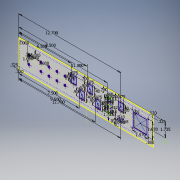
# Autodesk Inventor part: nmt_frontpanel
Saved by Autodesk Inventor 2017 (Build 210142000, 142)
## iProperties
Created: 2017-02-06
Part Number: nmt_frontpanel
Material: Generic
Document SubType Name: Modeling
Designer: Zara
Density: 1 g/cm^3
Appearance: Default
Author: Zara
Autodesk Inventor part; units mm, degrees
ref_plane "YZ Plane" through (0, 0, 0) normal (1, 0, 0) x (0, 1, 0)
ref_plane "XZ Plane" through (0, 0, 0) normal (0, 1, 0) x (-1, 0, 0)
ref_plane "XY Plane" through (0, 0, 0) normal (0, 0, 1) x (1, 0, 0)
sketch "Sketch1" plane through (0, 0, 0) normal (0, 0, 1) x (1, 0, 0)
  line L0 (-212.471, -44.069) -> (212.471, -44.069)
  line L1 (212.471, -44.069) -> (212.471, 44.069)
  line L2 (212.471, 44.069) -> (-212.471, 44.069)
  line L3 (-212.471, 44.069) -> (-212.471, -44.069)
  line L4 (-212.471, -44.069) -> (212.471, 44.069) construction
  line L5 (212.471, -44.069) -> (-212.471, 44.069) construction
  point P0 (0, 0)
  dimension "d0" = 424.942
  dimension "d1" = 88.138
  constraints: 12 end point, 2 midpoint, 2 parallel, 1 horizontal, 1 perpendicular
  measures "d0" distance of L1.end L2.end
  measures "d1" distance of L0.end L1.end
extrude "Extrusion1" add sketch "Sketch1" along normal blind 1.651
sketch "SMA" plane through (0, 0, 1.651) normal (0, 0, 1) x (1, 0, 0)
  line L0 (-209.423, -35.814) -> (209.423, -35.814) construction
  line L1 (209.423, -35.814) -> (209.423, 35.814) construction
  line L2 (209.423, 35.814) -> (-209.423, 35.814) construction
  line L3 (-209.423, 35.814) -> (-209.423, -35.814) construction
  line L4 (212.471, 44.069) -> (-212.471, 44.069) construction
  line L5 (212.471, -44.069) -> (212.471, 44.069) construction
  line L6 (-212.471, 44.069) -> (-212.471, -44.069) projected
  line L7 (-212.471, -44.069) -> (212.471, -44.069) projected
  line L8 (-222.5982, 0) -> (228.0899, 0) construction
  line L9 (0, 79.8165) -> (0, -88.5526) construction
  line L10 (-181.2798, 19.5533) -> (-181.2798, 0.2592) construction
  line L11 (-189.2532, 10.414) -> (-170.7489, 10.414) construction
  arc A0 (-184.023, 8.669) -> (-184.023, 12.159) centre (-181.2798, 10.414) ccw
  line L12 (-184.023, 12.159) -> (-184.023, 8.669)
  line L13 (-145.923, 12.159) -> (-145.923, 8.669)
  arc A1 (-145.923, 8.669) -> (-145.923, 12.159) centre (-143.1798, 10.414) ccw
  line L14 (-184.023, -13.241) -> (-184.023, -16.731)
  arc A2 (-184.023, -16.731) -> (-184.023, -13.241) centre (-181.2798, -14.986) ccw
  line L15 (-145.923, -13.241) -> (-145.923, -16.731)
  arc A3 (-145.923, -16.731) -> (-145.923, -13.241) centre (-143.1798, -14.986) ccw
  line L16 (-120.523, 12.159) -> (-120.523, 8.669)
  arc A4 (-120.523, 8.669) -> (-120.523, 12.159) centre (-117.7798, 10.414) ccw
  arc A5 (-120.523, -16.731) -> (-120.523, -13.241) centre (-117.7798, -14.986) ccw
  line L17 (-120.523, -13.241) -> (-120.523, -16.731)
  line L18 (-95.123, 12.159) -> (-95.123, 8.669)
  arc A6 (-95.123, 8.669) -> (-95.123, 12.159) centre (-92.3798, 10.414) ccw
  arc A7 (-95.123, -16.731) -> (-95.123, -13.241) centre (-92.3798, -14.986) ccw
  line L19 (-95.123, -13.241) -> (-95.123, -16.731)
  line L20 (-69.723, 12.159) -> (-69.723, 8.669)
  arc A8 (-69.723, 8.669) -> (-69.723, 12.159) centre (-66.9798, 10.414) ccw
  arc A9 (-69.723, -16.731) -> (-69.723, -13.241) centre (-66.9798, -14.986) ccw
  line L21 (-69.723, -13.241) -> (-69.723, -16.731)
  point P0 (0, 0)
  point P1 (-178.0286, 10.414)
  point P2 (-139.9286, 10.414)
  point P3 (-178.0286, -14.986)
  point P4 (-139.9286, -14.986)
  point P5 (-114.5286, 10.414)
  point P6 (-114.5286, -14.986)
  point P7 (-89.1286, 10.414)
  point P8 (-89.1286, -14.986)
  point P9 (-63.7286, 10.414)
  point P10 (-63.7286, -14.986)
  point P11 (-63.7286, -14.986)
  dimension "d4" = 8.255
  dimension "d5" = 3.048
  dimension "d7" = 8.255
  dimension "d8" = 3.048
  dimension "d11" = 6.5024
  dimension "d12" = 5.9944
  dimension "d13" = 25.4
  dimension "d14" = 25.4
  dimension "d17" = 38.1
  dimension "d20" = 25.4
  dimension "d25" = 25.4
  constraints: 36 end point, 30 point on circle, 10 centre point, 5 horizontal, 4 vertical, 3 point on line, 2 parallel, 1 coincident, 1 perpendicular, 54 other
  measures "d4" distance between parallel lines of L4 L2
  measures "d5" distance between parallel lines of L5 L1
  measures "d7" distance between parallel lines of L7 L0
  measures "d8" distance between parallel lines of L3 L6
  measures "d11" diameter of A0
  measures "d12" distance from line of point (-178.029, 10.414) L12
  measures "d13" distance between parallel lines of L3 L12
  measures "d14" distance from line of L2 A0.centre
  measures "d17" distance of L12.start L13.start
  measures "d20" distance of L12.start L14.start
  measures "d25" distance of L13.start L16.start
sketch "airflow" plane through (0, 0, 1.651) normal (0, 0, 1) x (1, 0, 0)
  line L0 (146.685, -25.019) -> (196.723, -25.019) construction
  line L1 (196.723, -25.019) -> (196.723, 25.019) construction
  line L2 (196.723, 25.019) -> (146.685, 25.019) construction
  line L3 (146.685, 25.019) -> (146.685, -25.019) construction
  line L4 (146.685, -25.019) -> (196.723, 25.019) construction
  line L5 (196.723, -25.019) -> (146.685, 25.019) construction
  line L6 (209.423, -35.814) -> (209.423, 35.814) construction
  line L7 (209.423, 35.814) -> (-209.423, 35.814) construction
  line L8 (-209.423, -35.814) -> (209.423, -35.814) construction
  line L9 (-209.423, 35.814) -> (-209.423, -35.814) construction
  line L10 (-212.471, -44.069) -> (212.471, -44.069) projected
  line L11 (212.471, -44.069) -> (212.471, 44.069) projected
  line L12 (212.471, 44.069) -> (-212.471, 44.069) projected
  line L13 (-212.471, 44.069) -> (-212.471, -44.069) projected
  line L14 (150.6195, -21.0845) -> (192.7885, -21.0845)
  line L15 (192.7885, -21.0845) -> (192.7885, 21.0845)
  line L16 (192.7885, 21.0845) -> (150.6195, 21.0845)
  line L17 (150.6195, 21.0845) -> (150.6195, -21.0845)
  line L18 (150.6195, -21.0845) -> (192.7885, 21.0845) construction
  line L19 (192.7885, -21.0845) -> (150.6195, 21.0845) construction
  point P0 (171.704, 0)
  point P1 (252.5868, -10.4776)
  dimension "d30" = 50.038
  dimension "d31" = 50.038
  dimension "d32" = 12.7
  dimension "d218" = 3.9345
  dimension "d229" = 44.069
  constraints: 24 end point, 4 coincident, 4 midpoint, 4 parallel, 2 horizontal, 2 perpendicular, 1 point on line
  measures "d30" distance of L0.end L1.end
  measures "d31" distance of L0.start L0.end
  measures "d32" distance between parallel lines of L1 L6
  measures "d218" distance between parallel lines of L2 L16
  measures "d229" distance from line of L12 point (171.704, 0)
sketch "Dsub25" plane through (0, 0, 1.651) normal (0, 0, 1) x (1, 0, 0)
  line L0 (78.613, 20.0279) -> (78.613, -20.0279)
  line L1 (66.929, 18.4404) -> (66.929, -18.4404)
  arc A0 (76.1166, -22.0536) -> (78.613, -20.0279) centre (76.5429, -20.0279) ccw
  arc A1 (66.929, -18.4404) -> (68.5728, -20.4661) centre (68.9991, -18.4404) ccw
  arc A2 (78.613, 20.0279) -> (76.1166, 22.0536) centre (76.5429, 20.0279) ccw
  arc A3 (68.5728, 20.4661) -> (66.929, 18.4404) centre (68.9991, 18.4404) ccw
  line L2 (49.6457, 0) -> (87.8983, 0) construction
  line L3 (-212.471, -44.069) -> (212.471, -44.069) construction
  line L4 (72.771, 23.5839) -> (72.771, -23.5839) construction
  line L5 (76.1166, 22.0536) -> (68.5728, 20.4661)
  line L6 (76.1166, -22.0536) -> (68.5728, -20.4661)
  line L7 (-212.471, 44.069) -> (-212.471, -44.069) projected
  point P0 (0, 0)
  point P1 (78.613, 0)
  point P2 (66.929, 0)
  point P3 (72.771, 0)
  point P4 (72.771, 21.3496)
  dimension "d46" = 47.1678
  dimension "d47" = 4.1402
  dimension "d48" = 4.1402
  dimension "d49" = 4.1402
  dimension "d50" = 4.1402
  dimension "d51" = 40.0558
  dimension "d52" = 36.8808
  dimension "d53" = 44.069
  dimension "d57" = 11.684
  dimension "d58" = 5.842
  dimension "d59" = 279.4
  dimension "d60" = 44.069
  constraints: 12 end point, 8 point on circle, 8 tangent, 4 centre point, 4 midpoint, 2 coincident, 2 point on line, 1 horizontal
  measures "d46" distance of L4.end L4.start
  measures "d47" diameter of A0
  measures "d48" diameter of A2
  measures "d49" diameter of A3
  measures "d50" diameter of A1
  measures "d51" distance of A0.centre A2.centre
  measures "d52" distance of A1.centre A3.centre
  measures "d53" distance between parallel lines of L3 L2
  measures "d57" distance between parallel lines of L1 L0
  measures "d58" distance from line of L0 L4.start
  measures "d59" distance between parallel lines of L1 L7
  measures "d60" distance from line of L3 point (72.771, 0)
extrude "sma cutouts" cut sketch "SMA" against normal through all
hole "dsub25 holes" at (72.771, 23.5839, 1.651) at (72.771, -23.5839, 1.651) direction (0, 0, -1) diameter 2.9464 end through all
extrude "dsub25 cutout" cut sketch "Dsub25" against normal through all
sketch "rj45" plane through (0, 0, 1.651) normal (0, 0, 1) x (1, 0, 0)
  line L0 (-47.371, 3.429) -> (-30.226, 3.429)
  line L1 (-30.226, 3.429) -> (-30.226, 26.289)
  line L2 (-30.226, 26.289) -> (-47.371, 26.289)
  line L3 (-47.371, 26.289) -> (-47.371, 3.429)
  line L4 (-47.371, 3.429) -> (-30.226, 26.289) construction
  line L5 (-30.226, 3.429) -> (-47.371, 26.289) construction
  line L6 (-38.7985, 29.337) -> (-38.7985, 0.381) construction
  line L7 (-212.471, 44.069) -> (-212.471, -44.069) construction
  line L8 (212.471, 44.069) -> (-212.471, 44.069) construction
  line L9 (3.429, 3.429) -> (20.574, 3.429)
  line L10 (20.574, 3.429) -> (20.574, 26.289)
  line L11 (20.574, 26.289) -> (3.429, 26.289)
  line L12 (3.429, 26.289) -> (3.429, 3.429)
  line L13 (3.429, 3.429) -> (20.574, 26.289) construction
  line L14 (20.574, 3.429) -> (3.429, 26.289) construction
  line L15 (12.0015, 29.337) -> (12.0015, 0.381) construction
  line L16 (-21.971, -25.527) -> (-4.826, -25.527)
  line L17 (-4.826, -25.527) -> (-4.826, -2.667)
  line L18 (-4.826, -2.667) -> (-21.971, -2.667)
  line L19 (-21.971, -2.667) -> (-21.971, -25.527)
  line L20 (-21.971, -25.527) -> (-4.826, -2.667) construction
  line L21 (-4.826, -25.527) -> (-21.971, -2.667) construction
  line L22 (-13.3985, 0.381) -> (-13.3985, -28.575) construction
  line L23 (28.829, -25.527) -> (45.974, -25.527)
  line L24 (45.974, -25.527) -> (45.974, -2.667)
  line L25 (45.974, -2.667) -> (28.829, -2.667)
  line L26 (28.829, -2.667) -> (28.829, -25.527)
  line L27 (28.829, -25.527) -> (45.974, -2.667) construction
  line L28 (45.974, -25.527) -> (28.829, -2.667) construction
  line L29 (37.4015, 0.381) -> (37.4015, -28.575) construction
  line L30 (-212.471, -44.069) -> (212.471, -44.069) construction
  line L31 (-38.7985, 0.381) -> (62.2062, 0.381) construction
  point P0 (0, 0)
  point P1 (-38.7985, 14.859)
  point P2 (-38.7985, 14.859)
  point P3 (12.0015, 14.859)
  point P4 (12.0015, 14.859)
  point P5 (-13.3985, -14.097)
  point P6 (-13.3985, -14.097)
  point P7 (37.4015, -14.097)
  point P8 (37.4015, -14.097)
  dimension "d160" = 28.956
  dimension "d161" = 22.86
  dimension "d162" = 17.145
  dimension "d163" = 165.1
  dimension "d164" = 17.78
  dimension "d165" = 28.956
  dimension "d166" = 22.86
  dimension "d167" = 17.145
  dimension "d168" = 28.956
  dimension "d169" = 22.86
  dimension "d170" = 17.145
  dimension "d171" = 28.956
  dimension "d172" = 22.86
  dimension "d173" = 17.145
  dimension "d174" = 17.78
  dimension "d175" = 215.9
  dimension "d177" = 190.5
  dimension "d179" = 241.3
  constraints: 58 end point, 16 midpoint, 8 coincident, 8 parallel, 8 perpendicular, 5 horizontal, 2 point on line
  measures "d160" distance of L6.start L6.end
  measures "d161" distance of L2.end L0.start
  measures "d162" distance of L1.end L2.end
  measures "d163" distance between parallel lines of L7 L3
  measures "d164" distance between parallel lines of L8 L2
  measures "d165" distance of L15.start L15.end
  measures "d166" distance of L11.end L9.start
  measures "d167" distance of L10.end L11.end
  measures "d168" distance of L22.start L22.end
  measures "d169" distance of L18.end L16.start
  measures "d170" distance of L17.end L18.end
  measures "d171" distance of L29.start L29.end
  measures "d172" distance of L25.end L23.start
  measures "d173" distance of L24.end L25.end
  measures "d174" distance between parallel lines of L8 L11
  measures "d175" distance between parallel lines of L7 L12
  measures "d177" distance between parallel lines of L7 L19
  measures "d179" distance between parallel lines of L7 L26
hole "rj45 holes" at (-38.7985, 29.337, 1.651) at (-38.7985, 0.381, 1.651) at (12.0015, 0.381, 1.651) at (12.0015, 29.337, 1.651) at (-13.3985, -28.575, 1.651) at (-13.3985, 0.381, 1.651) at (37.4015, -28.575, 1.651) at (37.4015, 0.381, 1.651) direction (0, 0, -1) diameter 3.2766 end through all clearance for "Flat Head Machine Screw (82)" size "#4" standard "Ansi Unified Screw Threads"
extrude "rj45 cutouts" cut sketch "rj45" against normal blind 25.4
sketch "rj45 debug" plane through (0, 0, 1.651) normal (0, 0, 1) x (1, 0, 0)
  line L0 (101.5365, 3.429) -> (118.6815, 3.429)
  line L1 (118.6815, 3.429) -> (118.6815, 26.289)
  line L2 (118.6815, 26.289) -> (101.5365, 26.289)
  line L3 (101.5365, 26.289) -> (101.5365, 3.429)
  line L4 (101.5365, 3.429) -> (118.6815, 26.289) construction
  line L5 (118.6815, 3.429) -> (101.5365, 26.289) construction
  line L6 (110.109, 29.337) -> (110.109, 0.381) construction
  line L7 (-212.471, 44.069) -> (-212.471, -44.069) projected
  line L8 (212.471, 44.069) -> (-212.471, 44.069) projected
  point P0 (0, 0)
  point P1 (110.109, 14.859)
  point P2 (110.109, 14.859)
  dimension "d189" = 28.956
  dimension "d190" = 17.145
  dimension "d191" = 22.86
  dimension "d193" = 17.78
  dimension "d194" = 322.58
  constraints: 14 end point, 4 midpoint, 2 coincident, 2 parallel, 1 horizontal, 1 perpendicular, 1 vertical
  measures "d189" distance of L6.start L6.end
  measures "d190" distance of L1.end L2.end
  measures "d191" distance of L0.end L1.end
  measures "d193" distance between parallel lines of L8 L2
  measures "d194" distance from line of L7 point (110.109, 14.859)
hole "rj45 debug holes" at (110.109, 29.337, 1.651) at (110.109, 0.381, 1.651) direction (0, 0, -1) diameter 3.2766 end through all clearance for "Flat Head Machine Screw (82)" size "#4" standard "Ansi Unified Screw Threads"
extrude "rj45 debug cutout" cut sketch "rj45 debug" against normal blind 25.4
sketch "SC/SC" plane through (0, 0, 1.651) normal (0, 0, 1) x (1, 0, 0)
  line L0 (103.632, -16.1798) -> (116.586, -16.1798)
  line L1 (116.586, -16.1798) -> (116.586, -25.527)
  line L2 (116.586, -25.527) -> (103.632, -25.527)
  line L3 (103.632, -25.527) -> (103.632, -16.1798)
  line L4 (103.632, -16.1798) -> (116.586, -25.527) construction
  line L5 (116.586, -16.1798) -> (103.632, -25.527) construction
  line L6 (101.109, -20.8534) -> (119.109, -20.8534) construction
  line L7 (-212.471, 44.069) -> (-212.471, -44.069) projected
  line L8 (-212.471, -44.069) -> (212.471, -44.069) projected
  point P0 (0, 0)
  point P1 (110.109, -20.8534)
  point P2 (110.109, -20.8534)
  dimension "d204" = 12.954
  dimension "d205" = 9.3472
  dimension "d206" = 18
  dimension "d207" = 322.58
  dimension "d208" = 18.542
  constraints: 14 end point, 4 midpoint, 2 coincident, 2 horizontal, 2 parallel, 1 perpendicular
  measures "d204" distance of L0.start L0.end
  measures "d205" distance of L0.end L1.end
  measures "d206" distance of L6.start L6.end
  measures "d207" distance from line of L7 point (110.109, -20.853)
  measures "d208" distance between parallel lines of L2 L8
hole "SC/SC holes" at (101.109, -20.8534, 1.651) at (119.109, -20.8534, 1.651) direction (0, 0, -1) diameter 2.3876 end through all clearance for "Countersunk Flat Head Screw ISO 2009/7046" size "M2" standard "ISO"
extrude "SC/SC cutout" cut sketch "SC/SC" against normal blind 25.4
hole "airflow holes" at (146.685, 25.019, 1.651) at (196.723, 25.019, 1.651) at (196.723, -25.019, 1.651) at (146.685, -25.019, 1.651) direction (0, 0, -1) diameter 5.1054 end through all clearance for "Flat Head Machine Screw (82)" size "#10" standard "Ansi Unified Screw Threads"
extrude "airflow cutout" cut sketch "airflow" against normal through all contours L17 L16 L15 L14
body "Solid1"
